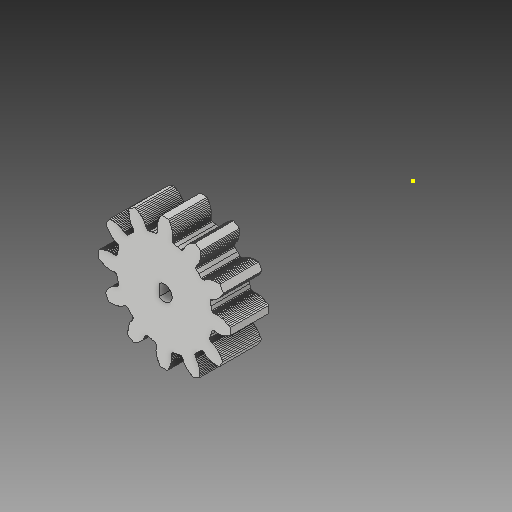
# Autodesk Inventor part: engranaje
Saved by Autodesk Inventor 2018.2 (Build 222227000, 227)
## iProperties
Created: 2016-05-04
Part Number: engranaje
Material: Genérico
Document SubType Name: Modeling
Designer: Usuario
Density: 1 g/cm^3
Appearance: Valor por defecto
Author: Usuario
Autodesk Inventor part; units mm, degrees
ref_plane "YZ Plane" through (0, 0, 0) normal (1, 0, 0) x (0, 1, 0)
ref_plane "XZ Plane" through (0, 0, 0) normal (0, 1, 0) x (-1, 0, 0)
ref_plane "XY Plane" through (0, 0, 0) normal (0, 0, 1) x (1, 0, 0)
sketch "Boceto1" plane through (0, 0, 0) normal (1, 0, 0) x (0, 1, 0)
  point P0 (0, 0)
extrude "Extrusión1" [suppressed]
sketch "Boceto2" plane through (10, 0, 0) normal (1, 0, 0) x (0, 0, -1)
  point P0 (0, 0)
sketch "Boceto3" plane through (10, 0, 0) normal (1, 0, 0) x (0, 0, -1)
  point P0 (0, 0)
sketch "Boceto4" plane through (10, 0, 0) normal (1, 0, 0) x (0, 0, -1)
  point P0 (0, 0)
sketch "Boceto5" plane through (10, 0, 0) normal (1, 0, 0) x (0, 0, -1)
  point P0 (0, 0)
sketch "Boceto6" plane through (10, 0, 0) normal (1, 0, 0) x (0, 0, -1)
  point P0 (0, 0)
sketch "Boceto7" plane through (10, 0, 0) normal (1, 0, 0) x (0, 0, -1)
  point P0 (0, 0)
sketch "Boceto8" plane through (0, 0, 0) normal (0, 0, 1) x (1, 0, 0)
  line L0 (-42.1833, -59.4872) -> (-42.3792, -59.5979)
  line L1 (-42.3792, -59.5979) -> (-42.4471, -59.6858)
  line L2 (-42.4471, -59.6858) -> (-42.4922, -59.7697)
  line L3 (-42.4922, -59.7697) -> (-42.5248, -59.8515)
  line L4 (-42.5248, -59.8515) -> (-42.5491, -59.932)
  line L5 (-42.5491, -59.932) -> (-42.567, -60.0115)
  line L6 (-42.567, -60.0115) -> (-42.5887, -60.1683)
  line L7 (-42.5887, -60.1683) -> (-42.5958, -60.3229)
  line L8 (-42.5958, -60.3229) -> (-42.5916, -60.476)
  line L9 (-42.5916, -60.476) -> (-42.5561, -60.7785)
  line L10 (-42.5561, -60.7785) -> (-42.5052, -61.0789)
  line L11 (-42.5052, -61.0789) -> (-42.5206, -61.3881)
  line L12 (-42.5206, -61.3881) -> (-42.5672, -61.7011)
  line L13 (-42.5672, -61.7011) -> (-42.6377, -62.0164)
  line L14 (-42.6377, -62.0164) -> (-42.7291, -62.3333)
  line L15 (-42.7291, -62.3333) -> (-42.8398, -62.6511)
  line L16 (-42.8398, -62.6511) -> (-42.9685, -62.9692)
  line L17 (-42.9685, -62.9692) -> (-43.1146, -63.2871)
  line L18 (-43.1146, -63.2871) -> (-43.2772, -63.6044)
  line L19 (-43.2772, -63.6044) -> (-43.4561, -63.9205)
  line L20 (-43.4561, -63.9205) -> (-43.6508, -64.2349)
  line L21 (-43.6508, -64.2349) -> (-45.4763, -64.2158)
  line L22 (-45.4763, -64.2158) -> (-45.6644, -63.8973)
  line L23 (-45.6644, -63.8973) -> (-45.8366, -63.5776)
  line L24 (-45.8366, -63.5776) -> (-45.9926, -63.257)
  line L25 (-45.9926, -63.257) -> (-46.1319, -62.9361)
  line L26 (-46.1319, -62.9361) -> (-46.2539, -62.6153)
  line L27 (-46.2539, -62.6153) -> (-46.3579, -62.2953)
  line L28 (-46.3579, -62.2953) -> (-46.4427, -61.9766)
  line L29 (-46.4427, -61.9766) -> (-46.5066, -61.6599)
  line L30 (-46.5066, -61.6599) -> (-46.5466, -61.346)
  line L31 (-46.5466, -61.346) -> (-46.5555, -61.0364)
  line L32 (-46.5555, -61.0364) -> (-46.4983, -60.7372)
  line L33 (-46.4983, -60.7372) -> (-46.4565, -60.4355)
  line L34 (-46.4565, -60.4355) -> (-46.4491, -60.2826)
  line L35 (-46.4491, -60.2826) -> (-46.453, -60.1278)
  line L36 (-46.453, -60.1278) -> (-46.4714, -59.9706)
  line L37 (-46.4714, -59.9706) -> (-46.4876, -59.8908)
  line L38 (-46.4876, -59.8908) -> (-46.5102, -59.8098)
  line L39 (-46.5102, -59.8098) -> (-46.5411, -59.7273)
  line L40 (-46.5411, -59.7273) -> (-46.5845, -59.6424)
  line L41 (-46.5845, -59.6424) -> (-46.6504, -59.5532)
  line L42 (-46.6504, -59.5532) -> (-46.844, -59.4384)
  line L43 (-46.844, -59.4384) -> (-47.7375, -59.2241)
  line L44 (-47.7375, -59.2241) -> (-48.6127, -58.9446)
  line L45 (-48.6127, -58.9446) -> (-48.8377, -58.9425)
  line L46 (-48.8377, -58.9425) -> (-48.9404, -58.9847)
  line L47 (-48.9404, -58.9847) -> (-49.0214, -59.0348)
  line L48 (-49.0214, -59.0348) -> (-49.0906, -59.0893)
  line L49 (-49.0906, -59.0893) -> (-49.1519, -59.1469)
  line L50 (-49.1519, -59.1469) -> (-49.2071, -59.2067)
  line L51 (-49.2071, -59.2067) -> (-49.3043, -59.3317)
  line L52 (-49.3043, -59.3317) -> (-49.3878, -59.4621)
  line L53 (-49.3878, -59.4621) -> (-49.4607, -59.5967)
  line L54 (-49.4607, -59.5967) -> (-49.5812, -59.8764)
  line L55 (-49.5812, -59.8764) -> (-49.6873, -60.162)
  line L56 (-49.6873, -60.162) -> (-49.8553, -60.4222)
  line L57 (-49.8553, -60.4222) -> (-50.0521, -60.6699)
  line L58 (-50.0521, -60.6699) -> (-50.2708, -60.9078)
  line L59 (-50.2708, -60.9078) -> (-50.5084, -61.1365)
  line L60 (-50.5084, -61.1365) -> (-50.7632, -61.3563)
  line L61 (-50.7632, -61.3563) -> (-51.0337, -61.5674)
  line L62 (-51.0337, -61.5674) -> (-51.3191, -61.7698)
  line L63 (-51.3191, -61.7698) -> (-51.6186, -61.9632)
  line L64 (-51.6186, -61.9632) -> (-51.9316, -62.1475)
  line L65 (-51.9316, -62.1475) -> (-52.2574, -62.3225)
  line L66 (-52.2574, -62.3225) -> (-53.8288, -61.3932)
  line L67 (-53.8288, -61.3932) -> (-53.8324, -61.0233)
  line L68 (-53.8324, -61.0233) -> (-53.8217, -60.6603)
  line L69 (-53.8217, -60.6603) -> (-53.7965, -60.3047)
  line L70 (-53.7965, -60.3047) -> (-53.7567, -59.9571)
  line L71 (-53.7567, -59.9571) -> (-53.702, -59.6183)
  line L72 (-53.702, -59.6183) -> (-53.6321, -59.2892)
  line L73 (-53.6321, -59.2892) -> (-53.5462, -58.9707)
  line L74 (-53.5462, -58.9707) -> (-53.4431, -58.6645)
  line L75 (-53.4431, -58.6645) -> (-53.3208, -58.3727)
  line L76 (-53.3208, -58.3727) -> (-53.1737, -58.1002)
  line L77 (-53.1737, -58.1002) -> (-52.9746, -57.8696)
  line L78 (-52.9746, -57.8696) -> (-52.7875, -57.6293)
  line L79 (-52.7875, -57.6293) -> (-52.7046, -57.5005)
  line L80 (-52.7046, -57.5005) -> (-52.6306, -57.3645)
  line L81 (-52.6306, -57.3645) -> (-52.5679, -57.2192)
  line L82 (-52.5679, -57.2192) -> (-52.5421, -57.1419)
  line L83 (-52.5421, -57.1419) -> (-52.5212, -57.0605)
  line L84 (-52.5212, -57.0605) -> (-52.5067, -56.9736)
  line L85 (-52.5067, -56.9736) -> (-52.5018, -56.8784)
  line L86 (-52.5018, -56.8784) -> (-52.5143, -56.7682)
  line L87 (-52.5143, -56.7682) -> (-52.6246, -56.572)
  line L88 (-52.6246, -56.572) -> (-53.2912, -55.9397)
  line L89 (-53.2912, -55.9397) -> (-53.9094, -55.26)
  line L90 (-53.9094, -55.26) -> (-54.1032, -55.1456)
  line L91 (-54.1032, -55.1456) -> (-54.2133, -55.1308)
  line L92 (-54.2133, -55.1308) -> (-54.3085, -55.1337)
  line L93 (-54.3085, -55.1337) -> (-54.3957, -55.1463)
  line L94 (-54.3957, -55.1463) -> (-54.4775, -55.1656)
  line L95 (-54.4775, -55.1656) -> (-54.5553, -55.1898)
  line L96 (-54.5553, -55.1898) -> (-54.7019, -55.2494)
  line L97 (-54.7019, -55.2494) -> (-54.8394, -55.3205)
  line L98 (-54.8394, -55.3205) -> (-54.9699, -55.4007)
  line L99 (-54.9699, -55.4007) -> (-55.2141, -55.5827)
  line L100 (-55.2141, -55.5827) -> (-55.4488, -55.777)
  line L101 (-55.4488, -55.777) -> (-55.7243, -55.9183)
  line L102 (-55.7243, -55.9183) -> (-56.0186, -56.0345)
  line L103 (-56.0186, -56.0345) -> (-56.3269, -56.1311)
  line L104 (-56.3269, -56.1311) -> (-56.6471, -56.2103)
  line L105 (-56.6471, -56.2103) -> (-56.9776, -56.2734)
  line L106 (-56.9776, -56.2734) -> (-57.3175, -56.3209)
  line L107 (-57.3175, -56.3209) -> (-57.6658, -56.3534)
  line L108 (-57.6658, -56.3534) -> (-58.0219, -56.3712)
  line L109 (-58.0219, -56.3712) -> (-58.3851, -56.3743)
  line L110 (-58.3851, -56.3743) -> (-58.7548, -56.363)
  line L111 (-58.7548, -56.363) -> (-59.651, -54.7724)
  line L112 (-59.651, -54.7724) -> (-59.4692, -54.4503)
  line L113 (-59.4692, -54.4503) -> (-59.2784, -54.1413)
  line L114 (-59.2784, -54.1413) -> (-59.0787, -53.8459)
  line L115 (-59.0787, -53.8459) -> (-58.8705, -53.5648)
  line L116 (-58.8705, -53.5648) -> (-58.6537, -53.2988)
  line L117 (-58.6537, -53.2988) -> (-58.4286, -53.0487)
  line L118 (-58.4286, -53.0487) -> (-58.195, -52.8159)
  line L119 (-58.195, -52.8159) -> (-57.9526, -52.6022)
  line L120 (-57.9526, -52.6022) -> (-57.7008, -52.4106)
  line L121 (-57.7008, -52.4106) -> (-57.4372, -52.2481)
  line L122 (-57.4372, -52.2481) -> (-57.1494, -52.1481)
  line L123 (-57.1494, -52.1481) -> (-56.8673, -52.0334)
  line L124 (-56.8673, -52.0334) -> (-56.7311, -51.9634)
  line L125 (-56.7311, -51.9634) -> (-56.599, -51.8826)
  line L126 (-56.599, -51.8826) -> (-56.472, -51.7881)
  line L127 (-56.472, -51.7881) -> (-56.411, -51.7341)
  line L128 (-56.411, -51.7341) -> (-56.3522, -51.6741)
  line L129 (-56.3522, -51.6741) -> (-56.2962, -51.606)
  line L130 (-56.2962, -51.606) -> (-56.2444, -51.5261)
  line L131 (-56.2444, -51.5261) -> (-56.2001, -51.4243)
  line L132 (-56.2001, -51.4243) -> (-56.1975, -51.1993)
  line L133 (-56.1975, -51.1993) -> (-56.4586, -50.3184)
  line L134 (-56.4586, -50.3184) -> (-56.6542, -49.4206)
  line L135 (-56.6542, -49.4206) -> (-56.7649, -49.2247)
  line L136 (-56.7649, -49.2247) -> (-56.8527, -49.1568)
  line L137 (-56.8527, -49.1568) -> (-56.9366, -49.1117)
  line L138 (-56.9366, -49.1117) -> (-57.0185, -49.0791)
  line L139 (-57.0185, -49.0791) -> (-57.0989, -49.0549)
  line L140 (-57.0989, -49.0549) -> (-57.1784, -49.0369)
  line L141 (-57.1784, -49.0369) -> (-57.3352, -49.0152)
  line L142 (-57.3352, -49.0152) -> (-57.4899, -49.0081)
  line L143 (-57.4899, -49.0081) -> (-57.6429, -49.0123)
  line L144 (-57.6429, -49.0123) -> (-57.9454, -49.0478)
  line L145 (-57.9454, -49.0478) -> (-58.2458, -49.0987)
  line L146 (-58.2458, -49.0987) -> (-58.5551, -49.0833)
  line L147 (-58.5551, -49.0833) -> (-58.868, -49.0368)
  line L148 (-58.868, -49.0368) -> (-59.1834, -48.9663)
  line L149 (-59.1834, -48.9663) -> (-59.5003, -48.8748)
  line L150 (-59.5003, -48.8748) -> (-59.818, -48.7641)
  line L151 (-59.818, -48.7641) -> (-60.1361, -48.6354)
  line L152 (-60.1361, -48.6354) -> (-60.4541, -48.4894)
  line L153 (-60.4541, -48.4894) -> (-60.7713, -48.3267)
  line L154 (-60.7713, -48.3267) -> (-61.0874, -48.1478)
  line L155 (-61.0874, -48.1478) -> (-61.4019, -47.9532)
  line L156 (-61.4019, -47.9532) -> (-61.3828, -46.1276)
  line L157 (-61.3828, -46.1276) -> (-61.0643, -45.9396)
  line L158 (-61.0643, -45.9396) -> (-60.7445, -45.7674)
  line L159 (-60.7445, -45.7674) -> (-60.4239, -45.6114)
  line L160 (-60.4239, -45.6114) -> (-60.103, -45.4721)
  line L161 (-60.103, -45.4721) -> (-59.7823, -45.35)
  line L162 (-59.7823, -45.35) -> (-59.4623, -45.246)
  line L163 (-59.4623, -45.246) -> (-59.1435, -45.1612)
  line L164 (-59.1435, -45.1612) -> (-58.8268, -45.0973)
  line L165 (-58.8268, -45.0973) -> (-58.5129, -45.0573)
  line L166 (-58.5129, -45.0573) -> (-58.2034, -45.0484)
  line L167 (-58.2034, -45.0484) -> (-57.9041, -45.1056)
  line L168 (-57.9041, -45.1056) -> (-57.6025, -45.1474)
  line L169 (-57.6025, -45.1474) -> (-57.4495, -45.1549)
  line L170 (-57.4495, -45.1549) -> (-57.2947, -45.1509)
  line L171 (-57.2947, -45.1509) -> (-57.1375, -45.1326)
  line L172 (-57.1375, -45.1326) -> (-57.0577, -45.1163)
  line L173 (-57.0577, -45.1163) -> (-56.9767, -45.0937)
  line L174 (-56.9767, -45.0937) -> (-56.8942, -45.0628)
  line L175 (-56.8942, -45.0628) -> (-56.8094, -45.0195)
  line L176 (-56.8094, -45.0195) -> (-56.7201, -44.9535)
  line L177 (-56.7201, -44.9535) -> (-56.6054, -44.7599)
  line L178 (-56.6054, -44.7599) -> (-56.3911, -43.8665)
  line L179 (-56.3911, -43.8665) -> (-56.1116, -42.9912)
  line L180 (-56.1116, -42.9912) -> (-56.1094, -42.7662)
  line L181 (-56.1094, -42.7662) -> (-56.1516, -42.6635)
  line L182 (-56.1516, -42.6635) -> (-56.2017, -42.5825)
  line L183 (-56.2017, -42.5825) -> (-56.2563, -42.5133)
  line L184 (-56.2563, -42.5133) -> (-56.3138, -42.4521)
  line L185 (-56.3138, -42.4521) -> (-56.3737, -42.3968)
  line L186 (-56.3737, -42.3968) -> (-56.4986, -42.2996)
  line L187 (-56.4986, -42.2996) -> (-56.629, -42.2161)
  line L188 (-56.629, -42.2161) -> (-56.7637, -42.1432)
  line L189 (-56.7637, -42.1432) -> (-57.0434, -42.0227)
  line L190 (-57.0434, -42.0227) -> (-57.329, -41.9166)
  line L191 (-57.329, -41.9166) -> (-57.5891, -41.7487)
  line L192 (-57.5891, -41.7487) -> (-57.8369, -41.5519)
  line L193 (-57.8369, -41.5519) -> (-58.0747, -41.3331)
  line L194 (-58.0747, -41.3331) -> (-58.3034, -41.0955)
  line L195 (-58.3034, -41.0955) -> (-58.5233, -40.8408)
  line L196 (-58.5233, -40.8408) -> (-58.7344, -40.5702)
  line L197 (-58.7344, -40.5702) -> (-58.9367, -40.2848)
  line L198 (-58.9367, -40.2848) -> (-59.1301, -39.9853)
  line L199 (-59.1301, -39.9853) -> (-59.3144, -39.6724)
  line L200 (-59.3144, -39.6724) -> (-59.4894, -39.3465)
  line L201 (-59.4894, -39.3465) -> (-58.5601, -37.7751)
  line L202 (-58.5601, -37.7751) -> (-58.1903, -37.7715)
  line L203 (-58.1903, -37.7715) -> (-57.8272, -37.7822)
  line L204 (-57.8272, -37.7822) -> (-57.4716, -37.8074)
  line L205 (-57.4716, -37.8074) -> (-57.124, -37.8472)
  line L206 (-57.124, -37.8472) -> (-56.7852, -37.9019)
  line L207 (-56.7852, -37.9019) -> (-56.4561, -37.9719)
  line L208 (-56.4561, -37.9719) -> (-56.1377, -38.0578)
  line L209 (-56.1377, -38.0578) -> (-55.8314, -38.1608)
  line L210 (-55.8314, -38.1608) -> (-55.5396, -38.2832)
  line L211 (-55.5396, -38.2832) -> (-55.2671, -38.4302)
  line L212 (-55.2671, -38.4302) -> (-55.0365, -38.6294)
  line L213 (-55.0365, -38.6294) -> (-54.7962, -38.8164)
  line L214 (-54.7962, -38.8164) -> (-54.6674, -38.8993)
  line L215 (-54.6674, -38.8993) -> (-54.5314, -38.9733)
  line L216 (-54.5314, -38.9733) -> (-54.3861, -39.036)
  line L217 (-54.3861, -39.036) -> (-54.3088, -39.0618)
  line L218 (-54.3088, -39.0618) -> (-54.2274, -39.0828)
  line L219 (-54.2274, -39.0828) -> (-54.1405, -39.0972)
  line L220 (-54.1405, -39.0972) -> (-54.0454, -39.1021)
  line L221 (-54.0454, -39.1021) -> (-53.9351, -39.0896)
  line L222 (-53.9351, -39.0896) -> (-53.7389, -38.9793)
  line L223 (-53.7389, -38.9793) -> (-53.1066, -38.3127)
  line L224 (-53.1066, -38.3127) -> (-52.4269, -37.6945)
  line L225 (-52.4269, -37.6945) -> (-52.3126, -37.5007)
  line L226 (-52.3126, -37.5007) -> (-52.2977, -37.3907)
  line L227 (-52.2977, -37.3907) -> (-52.3006, -37.2955)
  line L228 (-52.3006, -37.2955) -> (-52.3133, -37.2083)
  line L229 (-52.3133, -37.2083) -> (-52.3325, -37.1265)
  line L230 (-52.3325, -37.1265) -> (-52.3567, -37.0487)
  line L231 (-52.3567, -37.0487) -> (-52.4163, -36.902)
  line L232 (-52.4163, -36.902) -> (-52.4875, -36.7645)
  line L233 (-52.4875, -36.7645) -> (-52.5677, -36.6341)
  line L234 (-52.5677, -36.6341) -> (-52.7496, -36.3899)
  line L235 (-52.7496, -36.3899) -> (-52.9439, -36.1552)
  line L236 (-52.9439, -36.1552) -> (-53.0852, -35.8796)
  line L237 (-53.0852, -35.8796) -> (-53.2014, -35.5853)
  line L238 (-53.2014, -35.5853) -> (-53.298, -35.277)
  line L239 (-53.298, -35.277) -> (-53.3773, -34.9568)
  line L240 (-53.3773, -34.9568) -> (-53.4403, -34.6263)
  line L241 (-53.4403, -34.6263) -> (-53.4879, -34.2864)
  line L242 (-53.4879, -34.2864) -> (-53.5204, -33.9381)
  line L243 (-53.5204, -33.9381) -> (-53.5381, -33.582)
  line L244 (-53.5381, -33.582) -> (-53.5413, -33.2188)
  line L245 (-53.5413, -33.2188) -> (-53.5299, -32.8492)
  line L246 (-53.5299, -32.8492) -> (-51.9394, -31.9529)
  line L247 (-51.9394, -31.9529) -> (-51.6173, -32.1347)
  line L248 (-51.6173, -32.1347) -> (-51.3082, -32.3256)
  line L249 (-51.3082, -32.3256) -> (-51.0129, -32.5252)
  line L250 (-51.0129, -32.5252) -> (-50.7318, -32.7335)
  line L251 (-50.7318, -32.7335) -> (-50.4657, -32.9502)
  line L252 (-50.4657, -32.9502) -> (-50.2156, -33.1753)
  line L253 (-50.2156, -33.1753) -> (-49.9828, -33.409)
  line L254 (-49.9828, -33.409) -> (-49.7691, -33.6513)
  line L255 (-49.7691, -33.6513) -> (-49.5776, -33.9032)
  line L256 (-49.5776, -33.9032) -> (-49.4151, -34.1668)
  line L257 (-49.4151, -34.1668) -> (-49.315, -34.4545)
  line L258 (-49.315, -34.4545) -> (-49.2004, -34.7367)
  line L259 (-49.2004, -34.7367) -> (-49.1303, -34.8729)
  line L260 (-49.1303, -34.8729) -> (-49.0495, -35.005)
  line L261 (-49.0495, -35.005) -> (-48.955, -35.1319)
  line L262 (-48.955, -35.1319) -> (-48.901, -35.1929)
  line L263 (-48.901, -35.1929) -> (-48.841, -35.2517)
  line L264 (-48.841, -35.2517) -> (-48.773, -35.3077)
  line L265 (-48.773, -35.3077) -> (-48.693, -35.3595)
  line L266 (-48.693, -35.3595) -> (-48.5912, -35.4038)
  line L267 (-48.5912, -35.4038) -> (-48.3662, -35.4064)
  line L268 (-48.3662, -35.4064) -> (-47.4853, -35.1453)
  line L269 (-47.4853, -35.1453) -> (-46.5876, -34.9497)
  line L270 (-46.5876, -34.9497) -> (-46.3916, -34.8391)
  line L271 (-46.3916, -34.8391) -> (-46.3238, -34.7512)
  line L272 (-46.3238, -34.7512) -> (-46.2787, -34.6673)
  line L273 (-46.2787, -34.6673) -> (-46.246, -34.5855)
  line L274 (-46.246, -34.5855) -> (-46.2218, -34.505)
  line L275 (-46.2218, -34.505) -> (-46.2039, -34.4255)
  line L276 (-46.2039, -34.4255) -> (-46.1822, -34.2687)
  line L277 (-46.1822, -34.2687) -> (-46.175, -34.1141)
  line L278 (-46.175, -34.1141) -> (-46.1792, -33.961)
  line L279 (-46.1792, -33.961) -> (-46.2147, -33.6585)
  line L280 (-46.2147, -33.6585) -> (-46.2656, -33.3581)
  line L281 (-46.2656, -33.3581) -> (-46.2502, -33.0489)
  line L282 (-46.2502, -33.0489) -> (-46.2037, -32.7359)
  line L283 (-46.2037, -32.7359) -> (-46.1332, -32.4206)
  line L284 (-46.1332, -32.4206) -> (-46.0417, -32.1037)
  line L285 (-46.0417, -32.1037) -> (-45.9311, -31.7859)
  line L286 (-45.9311, -31.7859) -> (-45.8023, -31.4678)
  line L287 (-45.8023, -31.4678) -> (-45.6563, -31.1499)
  line L288 (-45.6563, -31.1499) -> (-45.4937, -30.8326)
  line L289 (-45.4937, -30.8326) -> (-45.3148, -30.5165)
  line L290 (-45.3148, -30.5165) -> (-45.1201, -30.2021)
  line L291 (-45.1201, -30.2021) -> (-43.2946, -30.2212)
  line L292 (-43.2946, -30.2212) -> (-43.1065, -30.5397)
  line L293 (-43.1065, -30.5397) -> (-42.9343, -30.8594)
  line L294 (-42.9343, -30.8594) -> (-42.7783, -31.18)
  line L295 (-42.7783, -31.18) -> (-42.639, -31.5009)
  line L296 (-42.639, -31.5009) -> (-42.5169, -31.8217)
  line L297 (-42.5169, -31.8217) -> (-42.413, -32.1417)
  line L298 (-42.413, -32.1417) -> (-42.3281, -32.4604)
  line L299 (-42.3281, -32.4604) -> (-42.2643, -32.7771)
  line L300 (-42.2643, -32.7771) -> (-42.2243, -33.091)
  line L301 (-42.2243, -33.091) -> (-42.2154, -33.4005)
  line L302 (-42.2154, -33.4005) -> (-42.2726, -33.6998)
  line L303 (-42.2726, -33.6998) -> (-42.3144, -34.0015)
  line L304 (-42.3144, -34.0015) -> (-42.3218, -34.1544)
  line L305 (-42.3218, -34.1544) -> (-42.3179, -34.3092)
  line L306 (-42.3179, -34.3092) -> (-42.2995, -34.4664)
  line L307 (-42.2995, -34.4664) -> (-42.2832, -34.5462)
  line L308 (-42.2832, -34.5462) -> (-42.2607, -34.6272)
  line L309 (-42.2607, -34.6272) -> (-42.2298, -34.7097)
  line L310 (-42.2298, -34.7097) -> (-42.1864, -34.7945)
  line L311 (-42.1864, -34.7945) -> (-42.1204, -34.8838)
  line L312 (-42.1204, -34.8838) -> (-41.9268, -34.9986)
  line L313 (-41.9268, -34.9986) -> (-41.0334, -35.2129)
  line L314 (-41.0334, -35.2129) -> (-40.1582, -35.4924)
  line L315 (-40.1582, -35.4924) -> (-39.9331, -35.4945)
  line L316 (-39.9331, -35.4945) -> (-39.8304, -35.4523)
  line L317 (-39.8304, -35.4523) -> (-39.7494, -35.4022)
  line L318 (-39.7494, -35.4022) -> (-39.6802, -35.3477)
  line L319 (-39.6802, -35.3477) -> (-39.619, -35.2901)
  line L320 (-39.619, -35.2901) -> (-39.5637, -35.2302)
  line L321 (-39.5637, -35.2302) -> (-39.4666, -35.1053)
  line L322 (-39.4666, -35.1053) -> (-39.3831, -34.9749)
  line L323 (-39.3831, -34.9749) -> (-39.3102, -34.8403)
  line L324 (-39.3102, -34.8403) -> (-39.1897, -34.5606)
  line L325 (-39.1897, -34.5606) -> (-39.0836, -34.275)
  line L326 (-39.0836, -34.275) -> (-38.9156, -34.0148)
  line L327 (-38.9156, -34.0148) -> (-38.7188, -33.767)
  line L328 (-38.7188, -33.767) -> (-38.5001, -33.5292)
  line L329 (-38.5001, -33.5292) -> (-38.2624, -33.3005)
  line L330 (-38.2624, -33.3005) -> (-38.0077, -33.0807)
  line L331 (-38.0077, -33.0807) -> (-37.7372, -32.8695)
  line L332 (-37.7372, -32.8695) -> (-37.4517, -32.6672)
  line L333 (-37.4517, -32.6672) -> (-37.1522, -32.4738)
  line L334 (-37.1522, -32.4738) -> (-36.8393, -32.2895)
  line L335 (-36.8393, -32.2895) -> (-36.5134, -32.1145)
  line L336 (-36.5134, -32.1145) -> (-34.9421, -33.0438)
  line L337 (-34.9421, -33.0438) -> (-34.9384, -33.4137)
  line L338 (-34.9384, -33.4137) -> (-34.9492, -33.7767)
  line L339 (-34.9492, -33.7767) -> (-34.9744, -34.1323)
  line L340 (-34.9744, -34.1323) -> (-35.0142, -34.4799)
  line L341 (-35.0142, -34.4799) -> (-35.0689, -34.8187)
  line L342 (-35.0689, -34.8187) -> (-35.1388, -35.1478)
  line L343 (-35.1388, -35.1478) -> (-35.2247, -35.4663)
  line L344 (-35.2247, -35.4663) -> (-35.3278, -35.7725)
  line L345 (-35.3278, -35.7725) -> (-35.4501, -36.0643)
  line L346 (-35.4501, -36.0643) -> (-35.5971, -36.3368)
  line L347 (-35.5971, -36.3368) -> (-35.7963, -36.5674)
  line L348 (-35.7963, -36.5674) -> (-35.9833, -36.8077)
  line L349 (-35.9833, -36.8077) -> (-36.0662, -36.9365)
  line L350 (-36.0662, -36.9365) -> (-36.1402, -37.0725)
  line L351 (-36.1402, -37.0725) -> (-36.2029, -37.2178)
  line L352 (-36.2029, -37.2178) -> (-36.2287, -37.2951)
  line L353 (-36.2287, -37.2951) -> (-36.2497, -37.3765)
  line L354 (-36.2497, -37.3765) -> (-36.2642, -37.4634)
  line L355 (-36.2642, -37.4634) -> (-36.269, -37.5585)
  line L356 (-36.269, -37.5585) -> (-36.2565, -37.6688)
  line L357 (-36.2565, -37.6688) -> (-36.1463, -37.865)
  line L358 (-36.1463, -37.865) -> (-35.4797, -38.4973)
  line L359 (-35.4797, -38.4973) -> (-34.8615, -39.177)
  line L360 (-34.8615, -39.177) -> (-34.6676, -39.2914)
  line L361 (-34.6676, -39.2914) -> (-34.5576, -39.3062)
  line L362 (-34.5576, -39.3062) -> (-34.4624, -39.3033)
  line L363 (-34.4624, -39.3033) -> (-34.3752, -39.2906)
  line L364 (-34.3752, -39.2906) -> (-34.2934, -39.2714)
  line L365 (-34.2934, -39.2714) -> (-34.2156, -39.2472)
  line L366 (-34.2156, -39.2472) -> (-34.069, -39.1876)
  line L367 (-34.069, -39.1876) -> (-33.9315, -39.1165)
  line L368 (-33.9315, -39.1165) -> (-33.801, -39.0363)
  line L369 (-33.801, -39.0363) -> (-33.5568, -38.8543)
  line L370 (-33.5568, -38.8543) -> (-33.3221, -38.66)
  line L371 (-33.3221, -38.66) -> (-33.0466, -38.5187)
  line L372 (-33.0466, -38.5187) -> (-32.7523, -38.4025)
  line L373 (-32.7523, -38.4025) -> (-32.4439, -38.3059)
  line L374 (-32.4439, -38.3059) -> (-32.1238, -38.2267)
  line L375 (-32.1238, -38.2267) -> (-31.7932, -38.1636)
  line L376 (-31.7932, -38.1636) -> (-31.4534, -38.1161)
  line L377 (-31.4534, -38.1161) -> (-31.1051, -38.0836)
  line L378 (-31.1051, -38.0836) -> (-30.749, -38.0658)
  line L379 (-30.749, -38.0658) -> (-30.3858, -38.0627)
  line L380 (-30.3858, -38.0627) -> (-30.0161, -38.074)
  line L381 (-30.0161, -38.074) -> (-29.1199, -39.6646)
  line L382 (-29.1199, -39.6646) -> (-29.3017, -39.9867)
  line L383 (-29.3017, -39.9867) -> (-29.4925, -40.2957)
  line L384 (-29.4925, -40.2957) -> (-29.6921, -40.5911)
  line L385 (-29.6921, -40.5911) -> (-29.9004, -40.8722)
  line L386 (-29.9004, -40.8722) -> (-30.1171, -41.1382)
  line L387 (-30.1171, -41.1382) -> (-30.3423, -41.3883)
  line L388 (-30.3423, -41.3883) -> (-30.5759, -41.6211)
  line L389 (-30.5759, -41.6211) -> (-30.8183, -41.8348)
  line L390 (-30.8183, -41.8348) -> (-31.0701, -42.0264)
  line L391 (-31.0701, -42.0264) -> (-31.3337, -42.1889)
  line L392 (-31.3337, -42.1889) -> (-31.6215, -42.2889)
  line L393 (-31.6215, -42.2889) -> (-31.9036, -42.4036)
  line L394 (-31.9036, -42.4036) -> (-32.0398, -42.4736)
  line L395 (-32.0398, -42.4736) -> (-32.1719, -42.5544)
  line L396 (-32.1719, -42.5544) -> (-32.2988, -42.6489)
  line L397 (-32.2988, -42.6489) -> (-32.3598, -42.7029)
  line L398 (-32.3598, -42.7029) -> (-32.4187, -42.7629)
  line L399 (-32.4187, -42.7629) -> (-32.4747, -42.831)
  line L400 (-32.4747, -42.831) -> (-32.5265, -42.9109)
  line L401 (-32.5265, -42.9109) -> (-32.5708, -43.0127)
  line L402 (-32.5708, -43.0127) -> (-32.5734, -43.2377)
  line L403 (-32.5734, -43.2377) -> (-32.3122, -44.1186)
  line L404 (-32.3122, -44.1186) -> (-32.1167, -45.0164)
  line L405 (-32.1167, -45.0164) -> (-32.006, -45.2123)
  line L406 (-32.006, -45.2123) -> (-31.9182, -45.2801)
  line L407 (-31.9182, -45.2801) -> (-31.8342, -45.3253)
  line L408 (-31.8342, -45.3253) -> (-31.7524, -45.3579)
  line L409 (-31.7524, -45.3579) -> (-31.6719, -45.3821)
  line L410 (-31.6719, -45.3821) -> (-31.5925, -45.4001)
  line L411 (-31.5925, -45.4001) -> (-31.4357, -45.4218)
  line L412 (-31.4357, -45.4218) -> (-31.281, -45.4289)
  line L413 (-31.281, -45.4289) -> (-31.1279, -45.4247)
  line L414 (-31.1279, -45.4247) -> (-30.8255, -45.3892)
  line L415 (-30.8255, -45.3892) -> (-30.5251, -45.3383)
  line L416 (-30.5251, -45.3383) -> (-30.2158, -45.3537)
  line L417 (-30.2158, -45.3537) -> (-29.9028, -45.4002)
  line L418 (-29.9028, -45.4002) -> (-29.5875, -45.4707)
  line L419 (-29.5875, -45.4707) -> (-29.2706, -45.5622)
  line L420 (-29.2706, -45.5622) -> (-28.9528, -45.6729)
  line L421 (-28.9528, -45.6729) -> (-28.6347, -45.8016)
  line L422 (-28.6347, -45.8016) -> (-28.3168, -45.9476)
  line L423 (-28.3168, -45.9476) -> (-27.9996, -46.1103)
  line L424 (-27.9996, -46.1103) -> (-27.6835, -46.2891)
  line L425 (-27.6835, -46.2891) -> (-27.369, -46.4838)
  line L426 (-27.369, -46.4838) -> (-27.3881, -48.3094)
  line L427 (-27.3881, -48.3094) -> (-27.7066, -48.4974)
  line L428 (-27.7066, -48.4974) -> (-28.0264, -48.6696)
  line L429 (-28.0264, -48.6696) -> (-28.347, -48.8256)
  line L430 (-28.347, -48.8256) -> (-28.6679, -48.9649)
  line L431 (-28.6679, -48.9649) -> (-28.9886, -49.087)
  line L432 (-28.9886, -49.087) -> (-29.3086, -49.191)
  line L433 (-29.3086, -49.191) -> (-29.6273, -49.2758)
  line L434 (-29.6273, -49.2758) -> (-29.9441, -49.3397)
  line L435 (-29.9441, -49.3397) -> (-30.258, -49.3796)
  line L436 (-30.258, -49.3796) -> (-30.5675, -49.3886)
  line L437 (-30.5675, -49.3886) -> (-30.8667, -49.3314)
  line L438 (-30.8667, -49.3314) -> (-31.1684, -49.2896)
  line L439 (-31.1684, -49.2896) -> (-31.3214, -49.2821)
  line L440 (-31.3214, -49.2821) -> (-31.4761, -49.286)
  line L441 (-31.4761, -49.286) -> (-31.6333, -49.3044)
  line L442 (-31.6333, -49.3044) -> (-31.7132, -49.3207)
  line L443 (-31.7132, -49.3207) -> (-31.7941, -49.3433)
  line L444 (-31.7941, -49.3433) -> (-31.8766, -49.3742)
  line L445 (-31.8766, -49.3742) -> (-31.9615, -49.4175)
  line L446 (-31.9615, -49.4175) -> (-32.0507, -49.4835)
  line L447 (-32.0507, -49.4835) -> (-32.1655, -49.6771)
  line L448 (-32.1655, -49.6771) -> (-32.3798, -50.5705)
  line L449 (-32.3798, -50.5705) -> (-32.6593, -51.4458)
  line L450 (-32.6593, -51.4458) -> (-32.6614, -51.6708)
  line L451 (-32.6614, -51.6708) -> (-32.6193, -51.7735)
  line L452 (-32.6193, -51.7735) -> (-32.5692, -51.8545)
  line L453 (-32.5692, -51.8545) -> (-32.5146, -51.9237)
  line L454 (-32.5146, -51.9237) -> (-32.457, -51.9849)
  line L455 (-32.457, -51.9849) -> (-32.3972, -52.0402)
  line L456 (-32.3972, -52.0402) -> (-32.2722, -52.1374)
  line L457 (-32.2722, -52.1374) -> (-32.1419, -52.2209)
  line L458 (-32.1419, -52.2209) -> (-32.0072, -52.2938)
  line L459 (-32.0072, -52.2938) -> (-31.7275, -52.4143)
  line L460 (-31.7275, -52.4143) -> (-31.4419, -52.5204)
  line L461 (-31.4419, -52.5204) -> (-31.1818, -52.6883)
  line L462 (-31.1818, -52.6883) -> (-30.934, -52.8851)
  line L463 (-30.934, -52.8851) -> (-30.6962, -53.1039)
  line L464 (-30.6962, -53.1039) -> (-30.4675, -53.3415)
  line L465 (-30.4675, -53.3415) -> (-30.2476, -53.5962)
  line L466 (-30.2476, -53.5962) -> (-30.0365, -53.8668)
  line L467 (-30.0365, -53.8668) -> (-29.8342, -54.1522)
  line L468 (-29.8342, -54.1522) -> (-29.6408, -54.4517)
  line L469 (-29.6408, -54.4517) -> (-29.4564, -54.7646)
  line L470 (-29.4564, -54.7646) -> (-29.2814, -55.0905)
  line L471 (-29.2814, -55.0905) -> (-30.2108, -56.6619)
  line L472 (-30.2108, -56.6619) -> (-30.5806, -56.6655)
  line L473 (-30.5806, -56.6655) -> (-30.9436, -56.6548)
  line L474 (-30.9436, -56.6548) -> (-31.2993, -56.6295)
  line L475 (-31.2993, -56.6295) -> (-31.6468, -56.5897)
  line L476 (-31.6468, -56.5897) -> (-31.9856, -56.5351)
  line L477 (-31.9856, -56.5351) -> (-32.3148, -56.4651)
  line L478 (-32.3148, -56.4651) -> (-32.6332, -56.3792)
  line L479 (-32.6332, -56.3792) -> (-32.9394, -56.2762)
  line L480 (-32.9394, -56.2762) -> (-33.2313, -56.1538)
  line L481 (-33.2313, -56.1538) -> (-33.5038, -56.0068)
  line L482 (-33.5038, -56.0068) -> (-33.7343, -55.8076)
  line L483 (-33.7343, -55.8076) -> (-33.9747, -55.6206)
  line L484 (-33.9747, -55.6206) -> (-34.1034, -55.5377)
  line L485 (-34.1034, -55.5377) -> (-34.2394, -55.4637)
  line L486 (-34.2394, -55.4637) -> (-34.3848, -55.401)
  line L487 (-34.3848, -55.401) -> (-34.462, -55.3752)
  line L488 (-34.462, -55.3752) -> (-34.5434, -55.3542)
  line L489 (-34.5434, -55.3542) -> (-34.6303, -55.3398)
  line L490 (-34.6303, -55.3398) -> (-34.7255, -55.3349)
  line L491 (-34.7255, -55.3349) -> (-34.8358, -55.3474)
  line L492 (-34.8358, -55.3474) -> (-35.032, -55.4577)
  line L493 (-35.032, -55.4577) -> (-35.6643, -56.1243)
  line L494 (-35.6643, -56.1243) -> (-36.344, -56.7425)
  line L495 (-36.344, -56.7425) -> (-36.4583, -56.9363)
  line L496 (-36.4583, -56.9363) -> (-36.4731, -57.0463)
  line L497 (-36.4731, -57.0463) -> (-36.4702, -57.1415)
  line L498 (-36.4702, -57.1415) -> (-36.4576, -57.2287)
  line L499 (-36.4576, -57.2287) -> (-36.4384, -57.3105)
  line L500 (-36.4384, -57.3105) -> (-36.4142, -57.3883)
  line L501 (-36.4142, -57.3883) -> (-36.3545, -57.535)
  line L502 (-36.3545, -57.535) -> (-36.2834, -57.6725)
  line L503 (-36.2834, -57.6725) -> (-36.2032, -57.8029)
  line L504 (-36.2032, -57.8029) -> (-36.0212, -58.0471)
  line L505 (-36.0212, -58.0471) -> (-35.8269, -58.2818)
  line L506 (-35.8269, -58.2818) -> (-35.6856, -58.5573)
  line L507 (-35.6856, -58.5573) -> (-35.5695, -58.8517)
  line L508 (-35.5695, -58.8517) -> (-35.4729, -59.16)
  line L509 (-35.4729, -59.16) -> (-35.3936, -59.4802)
  line L510 (-35.3936, -59.4802) -> (-35.3306, -59.8107)
  line L511 (-35.3306, -59.8107) -> (-35.283, -60.1506)
  line L512 (-35.283, -60.1506) -> (-35.2505, -60.4989)
  line L513 (-35.2505, -60.4989) -> (-35.2328, -60.855)
  line L514 (-35.2328, -60.855) -> (-35.2296, -61.2181)
  line L515 (-35.2296, -61.2181) -> (-35.241, -61.5878)
  line L516 (-35.241, -61.5878) -> (-36.8315, -62.484)
  line L517 (-36.8315, -62.484) -> (-37.1536, -62.3023)
  line L518 (-37.1536, -62.3023) -> (-37.4626, -62.1114)
  line L519 (-37.4626, -62.1114) -> (-37.758, -61.9118)
  line L520 (-37.758, -61.9118) -> (-38.0391, -61.7035)
  line L521 (-38.0391, -61.7035) -> (-38.3052, -61.4868)
  line L522 (-38.3052, -61.4868) -> (-38.5552, -61.2616)
  line L523 (-38.5552, -61.2616) -> (-38.7881, -61.028)
  line L524 (-38.7881, -61.028) -> (-39.0018, -60.7857)
  line L525 (-39.0018, -60.7857) -> (-39.1933, -60.5338)
  line L526 (-39.1933, -60.5338) -> (-39.3558, -60.2702)
  line L527 (-39.3558, -60.2702) -> (-39.4559, -59.9825)
  line L528 (-39.4559, -59.9825) -> (-39.5705, -59.7003)
  line L529 (-39.5705, -59.7003) -> (-39.6406, -59.5641)
  line L530 (-39.6406, -59.5641) -> (-39.7213, -59.4321)
  line L531 (-39.7213, -59.4321) -> (-39.8159, -59.3051)
  line L532 (-39.8159, -59.3051) -> (-39.8699, -59.2441)
  line L533 (-39.8699, -59.2441) -> (-39.9299, -59.1853)
  line L534 (-39.9299, -59.1853) -> (-39.9979, -59.1293)
  line L535 (-39.9979, -59.1293) -> (-40.0779, -59.0775)
  line L536 (-40.0779, -59.0775) -> (-40.1796, -59.0332)
  line L537 (-40.1796, -59.0332) -> (-40.4047, -59.0306)
  line L538 (-40.4047, -59.0306) -> (-41.2856, -59.2917)
  line L539 (-41.2856, -59.2917) -> (-42.1833, -59.4872)
  arc A0 (-45.7083, -48.7185) -> (-45.7083, -45.7185) centre (-44.3854, -47.2185) ccw
  line L540 (-45.7083, -48.7185) -> (-45.7083, -45.7185)
  constraints: 1082 end point, 2 point on circle, 1 centre point, 1 vertical
extrude "Extrusión2" add sketch "Boceto8" along normal blind 10
sketch "Boceto9" plane through (0, 0, 0) normal (0, 0, -1) x (-1, 0, 0)
  arc A0 (45.7083, -45.7185) -> (45.7083, -48.7185) centre (44.3854, -47.2185) ccw projected
  circle A1 centre (44.3854, -47.2185) radius 2
  point P0 (0, 0)
  constraints: 1 centre point, 1 coincident
extrude "Extrusión3" cut sketch "Boceto9" against normal blind 2
